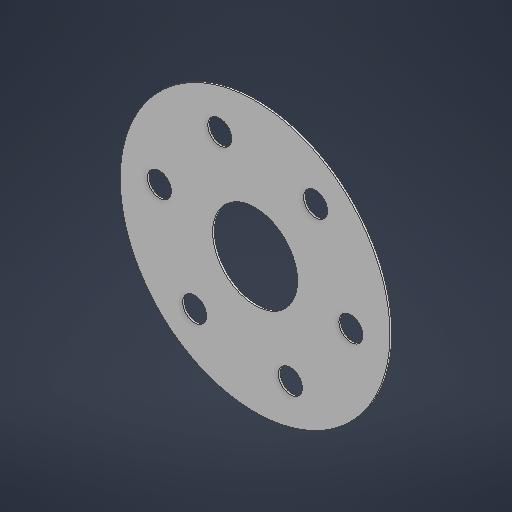
# Autodesk Inventor part: spool_spacer
Saved by Autodesk Inventor 2026.1 (Build 301233000, 233)
## iProperties
Created: 2026-04-28
Part Number: spool_spacer
Material: Generic
Document SubType Name: Modeling
Designer: aaron
Density: 1 g/cm^3
Appearance: Default
Author: aaron
Autodesk Inventor part; units mm, degrees
ref_plane "YZ Plane" through (0, 0, 0) normal (1, 0, 0) x (0, 1, 0)
ref_plane "XZ Plane" through (0, 0, 0) normal (0, 1, 0) x (-1, 0, 0)
ref_plane "XY Plane" through (0, 0, 0) normal (0, 0, 1) x (1, 0, 0)
sketch "Sketch1" plane through (0, 0, 0) normal (0, 0, 1) x (1, 0, 0)
  circle A0 centre (0, 0) radius 24
  circle A1 centre (0, 0) radius 7.55
  dimension "d0" = 48
  dimension "d1" = 15.1
  constraints: 2 centre point, 2 coincident
  measures "d0" diameter of A0
  measures "d1" diameter of A1
extrude "Extrusion1" add sketch "Sketch1" along normal blind 0.32
sketch "Sketch2" plane through (0, 0, 0) normal (0, 0, -1) x (-1, 0, 0)
  circle A0 centre (-16.5319, -11.256) radius 2.05 projected
  circle A1 centre (-19.649, 3.7306) radius 2.05 projected
  circle A2 centre (-17.0544, -2.5903) radius 1.65 projected
  circle A3 centre (-6.284, -16.0647) radius 1.65 projected
  circle A4 centre (-6.284, -16.0647) radius 1.65
  circle A5 centre (-6.284, -16.0647) radius 2.125
  circle A6 centre (10.7704, -13.4744) radius 2.125
  circle A7 centre (17.0544, 2.5903) radius 2.125
  circle A8 centre (6.284, 16.0647) radius 2.125
  circle A9 centre (-10.7704, 13.4744) radius 2.125
  circle A10 centre (-17.0544, -2.5903) radius 2.125
  point P0 (0, 0)
  dimension "d4" = 4.25
  dimension "d7" = 360
  constraints: 7 centre point, 2 coincident, 1 concentric, 13 other
  measures "d4" diameter of A5
extrude "Extrusion2" cut sketch "Sketch2" against normal through all contours A2 | A3 | A5 | A6 | A7 | A8 | A9 | A10
body "Solid1"
